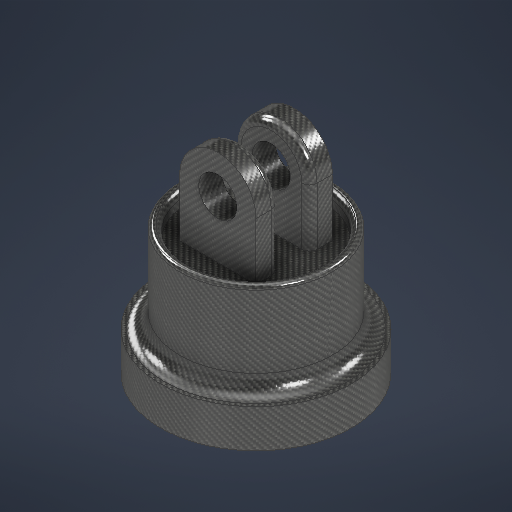
# Autodesk Inventor part: HANDBASE1
Saved by Autodesk Inventor 2027.1 (Build 311270010, 270A)
## iProperties
Created: 2026-08-27
Part Number: HANDBASE1
Material: Generic
Document SubType Name: Modeling
Designer: RIDDHIMAN
Density: 1 g/cm^3
Appearance: Default
Author: RIDDHIMAN
Autodesk Inventor part; units mm, degrees
ref_plane "YZ Plane" through (0, 0, 0) normal (1, 0, 0) x (0, 1, 0)
ref_plane "XZ Plane" through (0, 0, 0) normal (0, 1, 0) x (-1, 0, 0)
ref_plane "XY Plane" through (0, 0, 0) normal (0, 0, 1) x (1, 0, 0)
sketch "Sketch1" plane through (0, 0, 0) normal (0, 1, 0) x (-1, 0, 0)
  circle A0 centre (0, 0) radius 100
  dimension "d0" = 200
  constraints: 1 centre point, 1 coincident
  measures "d0" diameter of A0
extrude "Extrusion1" add sketch "Sketch1" along normal blind 120
sketch "Sketch2" plane through (0, 0, 0) normal (0, -1, 0) x (1, 0, 0)
  line L0 (125, 125) -> (-125, 125)
  line L1 (-125, 125) -> (-125, -125)
  line L2 (-125, -125) -> (125, -125)
  line L3 (125, -125) -> (125, 125)
  line L4 (125, 125) -> (-125, -125) construction
  line L5 (-125, 125) -> (125, -125) construction
  point P0 (0, 0)
  dimension "d3" = 250
  dimension "d4" = 250
  constraints: 12 end point, 2 midpoint, 2 parallel, 1 horizontal, 1 perpendicular
  measures "d3" distance of L2.end L1.end
  measures "d4" distance of L1.end L0.end
extrude "Extrusion2" add sketch "Sketch2" along normal blind 50
fillet "Fillet1" radius 20 1 edges at (100, 0, 0)
sketch "Sketch3" plane through (0, 120, 0) normal (0, 1, 0) x (1, 0, 0)
  circle A0 centre (0, 0) radius 87.5
  dimension "d8" = 175
  constraints: 1 centre point, 1 coincident
  measures "d8" diameter of A0
extrude "Extrusion3" cut sketch "Sketch3" against normal blind 20
fillet "Fillet2" radius 10 1 edges at (-87.5, 120, 0)
sketch "Sketch4" plane through (0, 100, 0) normal (0, 1, 0) x (1, 0, 0)
  line L0 (-50, -50) -> (50, -50)
  line L1 (50, -50) -> (50, 50)
  line L2 (50, 50) -> (-50, 50)
  line L3 (-50, 50) -> (-50, -50)
  line L4 (-50, -50) -> (50, 50) construction
  line L5 (50, -50) -> (-50, 50) construction
  line L6 (-50, -50) -> (50, -50)
  line L7 (50, -50) -> (50, -20)
  line L8 (50, -20) -> (-50, -20)
  line L9 (-50, -20) -> (-50, -50)
  line L10 (-50, 50) -> (50, 50)
  line L11 (50, 50) -> (50, 20)
  line L12 (50, 20) -> (-50, 20)
  line L13 (-50, 20) -> (-50, 50)
  point P0 (0, 0)
  dimension "d12" = 100
  dimension "d13" = 100
  dimension "d14" = 30
  dimension "d15" = 30
  constraints: 28 end point, 6 parallel, 3 horizontal, 3 perpendicular, 2 midpoint, 2 point on line
  measures "d12" distance of L2.end L1.end
  measures "d13" distance of L1.end L0.end
  measures "d14" distance of L7.end L6.end
  measures "d15" distance of L10.end L11.end
extrude "Extrusion4" add sketch "Sketch4" along normal blind 125 contours L3 L8 L1 L0 | L3 L2 L1 L12
sketch "Sketch5" plane through (50, 100, -50) normal (0, 0, -1) x (-1, 0, 0)
  circle A0 centre (50, 75) radius 50
  line L0 (0, 0) -> (0, 125) projected
  line L1 (0, 75) -> (0, 125)
  line L2 (0, 125) -> (100, 125)
  line L3 (100, 125) -> (100, 75)
  circle A1 centre (50, 75) radius 25
  point P0 (50, -100)
  point P1 (50, 125)
  dimension "d18" = 50
  constraints: 6 end point, 2 centre point, 2 point on circle, 1 coincident, 1 perpendicular, 1 tangent, 1 vertical
  measures "d18" diameter of A1
extrude "Extrusion5" cut sketch "Sketch5" against normal blind 125 contours L0 L2 A0 | A0 L2 L3 | A1
fillet "Fillet3" radius 10 3 edges at (-50, 137.5, -20) (0, 225, -20) (50, 137.5, -20)
fillet "Fillet4" radius 10 3 edges at (0, 225, 20) (50, 137.5, 20) (-50, 137.5, 20)
fillet "Fillet5" radius 5 1 edges at (100, 120, 0)
fillet "Fillet6" radius 125 4 edges at (125, -25, 125) (125, -25, -125) (-125, -25, 125) (-125, -25, -125)
sketch "Sketch6" plane through (0, -50, 0) normal (0, -1, 0) x (1, 0, 0)
  circle A0 centre (0, 0) radius 60
  dimension "d25" = 120
  constraints: 1 centre point, 1 coincident
  measures "d25" diameter of A0
extrude "Extrusion6" add sketch "Sketch6" along normal blind 10
body "Solid1"
